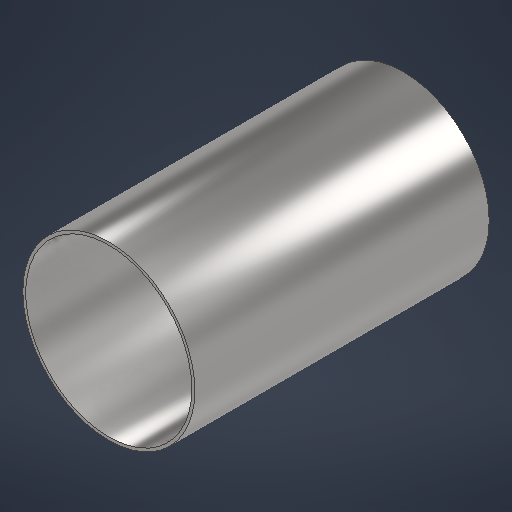
# Autodesk Inventor part: A
Saved by Autodesk Inventor 2025 (Build 290162000, 162)
## iProperties
RuleStatus: InUse
Created: 2024-06-07
Part Number: A
Material: 不鏽鋼
Document SubType Name: Modeling
Designer: a0976
Density: 8 g/cm^3
Appearance: 半拋光
Author: a0976
Autodesk Inventor part; units mm, degrees
ref_plane "YZ Plane" through (0, 0, 0) normal (1, 0, 0) x (0, 1, 0)
ref_plane "XZ Plane" through (0, 0, 0) normal (0, 1, 0) x (-1, 0, 0)
ref_plane "XY Plane" through (0, 0, 0) normal (0, 0, 1) x (1, 0, 0)
sketch "草圖1" plane through (0, 0, 0) normal (0, 0, 1) x (1, 0, 0)
  circle A0 centre (0, 0) radius 109.55
  line L0 (-94.8731, -54.775) -> (-98.1293, -56.655)
  line L1 (94.8731, -54.775) -> (98.1293, -56.655)
  line L2 (-117.81, 0) -> (117.81, 0) projected
  arc A1 (-98.1293, -56.655) -> (98.1293, -56.655) centre (0, 0) ccw
  circle A2 centre (0, 0) radius 105.79
  dimension "d0" = 219.1
  dimension "d4" = 120
  dimension "d5" = 30
  dimension "d6" = 30
  dimension "d7" = 3.76
  dimension "d12" = 3.76
  constraints: 4 end point, 4 point on circle, 3 centre point, 2 coincident
  measures "d0" diameter of A0
  measures "d4" angle of L1 L0
  measures "d5" angle of L2 L0
  measures "d6" angle of L2 L1
  measures "d7" radial gap between concentric circles of A1 A0
  measures "d12" radial gap between concentric circles of A0 A2
sketch "草圖2" plane through (0, 0, 0) normal (0, 0, 1) x (1, 0, 0)
  line L0 (-44.45, 0) -> (44.45, 0) construction
  line L1 (-50, -209.55) -> (50, -209.55)
  line L2 (0, -109.55) -> (-51.4901, -109.55) construction
  line L3 (0, -113.31) -> (0, -136.45) construction
  line L4 (-50, -201.55) -> (-50, -209.55)
  line L5 (50, -209.55) -> (50, -201.55)
  line L6 (-50, -201.55) -> (-2.75, -201.55)
  line L7 (2.75, -201.55) -> (50, -201.55)
  line L8 (-51.4901, -113.31) -> (60.072, -113.31)
  line L9 (-2.75, -201.55) -> (-2.75, -113.31)
  line L10 (2.75, -201.55) -> (2.75, -113.31)
  arc A0 (-98.1293, -56.655) -> (98.1293, -56.655) centre (0, 0) ccw projected
  circle A1 centre (0, 0) radius 109.55 projected
  point P0 (2.75, -209.55)
  point P1 (-2.75, -209.55)
  point P2 (2.75, -87.55)
  point P3 (-2.75, -87.55)
  dimension "d14" = 100
  dimension "d15" = 100
  dimension "d18" = 8
  dimension "d19" = 5.5
  dimension "d20" = 5.5
  dimension "d21" = 8
  dimension "d22" = 100
  constraints: 22 end point, 5 perpendicular, 4 point on line, 3 horizontal, 3 parallel, 1 point on circle, 1 symmetric about line, 1 vertical, 1 vertical alignment, 1 other
  measures "d14" distance from line of L2.start L1
  measures "d15" distance of L1.start L1.end
  measures "d18" distance between parallel lines of L1 L7
  measures "d19" distance between parallel lines of L9 L10
  measures "d20" diameter of L10 L3
  measures "d21" distance between parallel lines of L1 L6
  measures "d22" diameter of L5 L3
extrude "擠出4" add sketch "草圖1" along normal mid plane 375 contours A0 L2 A2 | A0 L2 A2
equation "\"d12\" = d7"
equation "\"d14\" = Hops"
equation "\"d15\" = Section_buttom_A"
equation "\"d18\" = Section_Top_thick"
equation "\"d19\" = Section_mid_thick"
equation "\"d20\" = Section_mid_thick"
equation "\"d21\" = d18"
equation "\"d22\" = d15"
equation "\"d25\" = 1.5 * Extra_Lops"
equation "\"Section_buttom_A\" = 100"
equation "\"Extra_Plate_B\" = 0"
equation "\"Section_mid_thick\" = 5.5"
equation "\"Section_Top_thick\" = 8"
equation "\"Section_front_gap\" = 35"
equation "\"Section_side_Gap\" = 25"
equation "\"Hops\" = 100"
equation "\"d17\" = Section_Top_thick"
equation "\"Extra_Lops\" = 250"
